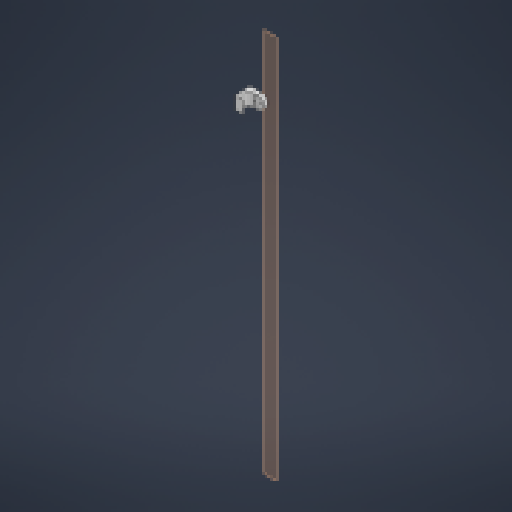
# Autodesk Inventor part: CNC-029-WireConduitHolder
Saved by Autodesk Inventor 2026.2 (Build 302298000, 298)
## iProperties
Created: 2026-06-28
Part Number: CNC-029-WireConduitHolder
Material: Generic
Document SubType Name: Modeling
Designer: Kenji
Density: 1 g/cm^3
Appearance: Default
Author: Kenji
Autodesk Inventor part; units mm, degrees
ref_plane "YZ Plane" through (0, 0, 0) normal (1, 0, 0) x (0, 1, 0)
ref_plane "XZ Plane" through (0, 0, 0) normal (0, 1, 0) x (-1, 0, 0)
ref_plane "Work Plane1" through (0, 0, 0) normal (0, 0, 1) x (1, 0, 0)
sketch "Sketch1" plane through (0, 0, 0) normal (0, 0, 1) x (1, 0, 0)
  line L0 (-0.508, 0) -> (-0.508, -400) projected
  line L1 (-5.768, 0) -> (-5.768, -400) projected
  circle A0 centre (-3.138, -50.8) radius 2.63
  line L2 (-13.138, 0) -> (-13.138, -400) projected
  circle A1 centre (-3.138, -50.8) radius 7.3925 construction
  line L3 (-3.138, -58.1925) -> (-15.838, -58.1925)
  line L4 (-15.838, -58.1925) -> (-15.838, -43.4075)
  line L5 (-15.838, -43.4075) -> (-3.138, -43.4075)
  arc A2 (-3.138, -58.1925) -> (-3.138, -43.4075) centre (-3.138, -50.8) ccw
  point P0 (0, 0)
  dimension "d0" = 5.26
  dimension "d1" = 10
  dimension "d2" = 4.7625
  dimension "d3" = 12.7
  dimension "d4" = 50.8
  constraints: 6 end point, 4 point on circle, 3 centre point, 3 tangent, 2 perpendicular, 1 horizontal
  measures "d0" diameter of A0
  measures "d1" distance from line of L2 A0.centre
  measures "d2" radial gap between concentric circles of A0 A1
  measures "d3" distance from line of L4 A0.centre
  measures "d4" vertical distance of L0.start A0.centre
extrude "Extrusion1" add sketch "Sketch1" along normal blind 8.2625 contours A2 L0 | L0 A0 L1 L5 A2 | L0 A2 L3 L1 A0 | L1 L3 L2 L5 | L2 L3 L4 L5
sketch "Sketch2" plane through (0, 0, 8.2625) normal (0, 0, 1) x (1, 0, 0)
  line L0 (-15.838, -43.4075) -> (-15.838, -58.1925) projected
  line L1 (-15.838, -58.1925) -> (-3.138, -58.1925) projected
  arc A0 (-3.138, -58.1925) -> (-3.138, -43.4075) centre (-3.138, -50.8) ccw projected
  line L2 (-3.138, -43.4075) -> (-15.838, -43.4075) projected
  circle A1 centre (-3.138, -50.8) radius 2.63 projected
  line L3 (-3.138, -43.4075) -> (-15.838, -43.4075) projected
  line L4 (-12.663, -43.4075) -> (-12.663, -58.1925)
  point P0 (0, 0)
  dimension "d7" = 3.175
  constraints: 2 end point, 2 point on line, 1 perpendicular
  measures "d7" distance between parallel lines of L0 L4
extrude "Extrusion2" add sketch "Sketch2" along normal blind 12.7 contours L2 L4 L1 L0
sketch "Sketch3" plane through (-15.838, -43.4075, 0) normal (0, 1, 0) x (1, 0, 0)
  circle A0 centre (9.525, -14.6125) radius 6.35 construction
  line L0 (12.7, -8.2625) -> (3.175, -8.2625) projected
  line L1 (3.175, -8.2625) -> (3.175, -20.9625) projected
  line L2 (3.175, -20.9625) -> (9.525, -20.9625)
  arc A1 (9.525, -8.2625) -> (9.525, -20.9625) centre (9.525, -14.6125) ccw
  point P0 (15.838, 0)
  point P1 (3.175, -14.6125)
  dimension "d10" = 12.7
  constraints: 4 point on circle, 4 tangent, 2 centre point, 2 end point, 1 concentric, 1 point on line
  measures "d10" diameter of A0
extrude "Extrusion3" add sketch "Sketch3" against normal up to surface (14.785 mm away)
fillet "Fillet1" radius 0.0247 1 edges at (-6.313, -50.8, 20.9625)
chamfer "Chamfer1" distance 0.7937 angle 45 2 edges at (-15.838, -50.8, 0) (-15.838, -50.8, 20.9625)
sketch "Sketch4" plane through (-3.138, -43.4075, 8.2625) normal (0, 1, 0) x (1, 0, 0)
  arc A0 (-3.175, 0) -> (-3.9641, -12.6508) centre (-3.175, -6.35) ccw projected
  arc A1 (-3.9641, -12.6508) -> (-2.6216, -12.6758) centre (-3.175, -6.35) ccw
  arc A2 (-3.9672, -12.7) -> (-3.9641, -12.6508) centre (-3.9672, -12.6753) ccw projected
  line L0 (-3.175, -6.35) -> (-2.6216, -12.6758) construction
  line L1 (-3.175, -6.35) -> (-3.175, -12.7) construction
  line L2 (-2.6216, -12.6758) -> (-2.6216, -14.2875)
  line L3 (-2.6216, -14.2875) -> (-12.7, -14.2875)
  line L4 (-11.9062, -12.7) -> (-12.7, -11.9062) projected
  line L5 (-12.7, -14.2875) -> (-12.7, -11.9062)
  line L6 (-11.9062, -12.7) -> (-3.9672, -12.7) projected
  point P0 (3.138, 8.2625)
  point P1 (-3.9425, -12.6768)
  dimension "d18" = 5
  dimension "d19" = 1.5875
  constraints: 10 end point, 6 point on circle, 2 vertical, 1 centre point, 1 horizontal, 1 perpendicular
  measures "d18" angle of L1 L0
  measures "d19" distance between parallel lines of L3 L6
extrude "Extrusion4" add sketch "Sketch4" against normal up to surface (14.785 mm away)
fillet "Fillet2" radius 0.3969 1 edges at (-5.7596, -50.8, 20.9383)
chamfer "Chamfer2" distance 0.3969 angle 45 2 edges at (-5.7596, -50.8, 22.55) (-15.838, -50.8, 22.55)
sketch "Sketch5" plane through (0, 0, 8.2625) normal (0, 0, 1) x (1, 0, 0)
  circle A0 centre (-3.138, -50.8) radius 2.63 projected
  circle A1 centre (-3.138, -50.8) radius 5
  point P0 (0, 0)
  dimension "d26" = 10
  constraints: 1 centre point, 1 coincident
  measures "d26" diameter of A1
extrude "Extrusion5" cut sketch "Sketch5" along normal mid plane 10
body "Solid1"
